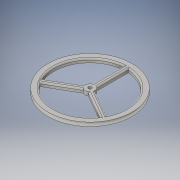
# Autodesk Inventor part: 3inwheel
Saved by Autodesk Inventor 2016 (Build 200138000, 138)
## iProperties
Created: 2018-05-30
Part Number: 3inwheel
Material: Generic
Document SubType Name: Modeling
Designer: Andrew
Density: 1 g/cm^3
Appearance: Default
Author: Andrew
Autodesk Inventor part; units mm, degrees
ref_plane "YZ Plane" through (0, 0, 0) normal (1, 0, 0) x (0, 1, 0)
ref_plane "XZ Plane" through (0, 0, 0) normal (0, 1, 0) x (-1, 0, 0)
ref_plane "XY Plane" through (0, 0, 0) normal (0, 0, 1) x (1, 0, 0)
sketch "Sketch1" plane through (0, 0, 0) normal (0, 0, 1) x (1, 0, 0)
  line L0 (1.778, -2.032) -> (44.45, -2.032)
  line L1 (44.45, 2.032) -> (1.778, 2.032)
  arc A0 (44.45, 2.032) -> (44.45, -2.032) centre (44.45, 0) ccw
  line L2 (0, -2.032) -> (0, 2.032)
  line L3 (1.778, -2.032) -> (1.778, 2.032)
  point P0 (0, 0)
  dimension "d3" = 1.778
  constraints: 8 end point, 2 parallel, 2 point on circle, 1 centre point, 1 horizontal
  measures "d3" distance between parallel lines of L2 L3
revolve "Revolution1" add sketch "Sketch1" angle 360 about axis through (0, -2.032, 0) along (0, 1, 0)
sketch "Sketch2" plane through (0, 2.032, 0) normal (0, 1, 0) x (1, 0, 0)
  line L0 (-2.54, 4.3994) -> (-2.54, 38.1)
  line L1 (2.54, 4.3994) -> (2.54, 38.1)
  circle A0 centre (0, 0) radius 1.778
  line L2 (-5.08, 0) -> (-34.2656, -16.8503)
  line L3 (-31.7256, -21.2497) -> (-2.54, -4.3994)
  line L4 (2.54, -4.3994) -> (31.7256, -21.0974)
  line L5 (34.2656, -16.8503) -> (5.08, 0)
  arc A1 (5.08, 0) -> (2.54, 4.3994) centre (0, 0) ccw
  arc A2 (-2.54, 4.3994) -> (-5.08, 0) centre (0, 0) ccw
  arc A3 (-2.54, -4.3994) -> (2.54, -4.3994) centre (0, 0) ccw
  arc A4 (34.1922, -16.8079) -> (2.54, 38.0152) centre (0, 0) ccw
  arc A5 (-2.54, 38.0152) -> (-34.1922, -16.8079) centre (0, 0) ccw
  arc A6 (-31.6522, -21.2073) -> (31.7256, -21.0974) centre (0, 0) ccw
  constraints: 12 end point, 12 point on circle, 7 centre point, 5 point on line, 2 coincident, 1 parallel
extrude "Extrusion1" cut sketch "Sketch2" against normal through all contours A2 L2 A5 L0 | L1 A4 L5 A1 | L3 A3 L4 A6
fillet "Fillet1" radius 1.524 1 edges at (-17.0961, 2.032, 12.8034)
fillet "Fillet4" radius 1.524 9 edges at (17.1328, 2.032, 12.7484) (19.6361, 2.032, 8.404) (2.54, 2.032, -21.2073) (-2.54, 2.032, -21.2073) (-32.0704, 2.032, 20.5693) (0.0661, 2.032, 38.0999) (-32.9956, 2.032, -19.05) (32.9956, 2.032, -19.05) (-19.6361, 2.032, 8.404)
body "Solid1"
